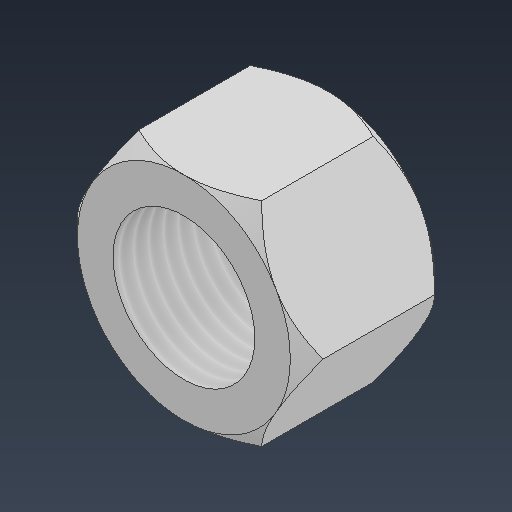
# Autodesk Inventor part: MCEN4000:T4
Saved by Autodesk Inventor 2021 (Build 250183000, 183)
## iProperties
Created: 2020-10-18
Part Number: MCEN4000:T4
Material: Generic
Document SubType Name: Modeling
Designer: Eugene Tang
Mass: 2.02151 g
Surface Area: 15.1772 cm^2
Volume: 2.02151 cm^3
Density: 1 g/cm^3
Appearance: Default
Description: NUT FASTENER
Author: Eugene Tang
Autodesk Inventor part; units mm, degrees
ref_plane "YZ Plane" through (0, 0, 0) normal (1, 0, 0) x (0, 1, 0)
ref_plane "XZ Plane" through (0, 0, 0) normal (0, 1, 0) x (-1, 0, 0)
ref_plane "XY Plane" through (0, 0, 0) normal (0, 0, 1) x (1, 0, 0)
sketch "Sketch1" plane through (0, 0, 0) normal (0, 0, 1) x (1, 0, 0)
  line L0 (10.3923, 0) -> (5.1962, -9)
  line L1 (5.1962, -9) -> (-5.1962, -9)
  line L2 (-5.1962, -9) -> (-10.3923, 0)
  line L3 (-10.3923, 0) -> (-5.1962, 9)
  line L4 (-5.1962, 9) -> (5.1962, 9)
  line L5 (5.1962, 9) -> (10.3923, 0)
  circle A0 centre (0, 0) radius 6
  dimension "d2" = 18
  dimension "d3" = 12
  constraints: 12 end point, 2 coincident, 1 centre point, 1 horizontal, 13 other
  measures "d2" distance between parallel lines of L3 L0
  measures "d3" diameter of A0
extrude "Extrusion2" add sketch "Sketch1" along normal blind 12.2
sketch "Sketch2" plane through (0, 0, 12.2) normal (0, 0, 1) x (1, 0, 0)
  circle A0 centre (0, 0) radius 6 construction
  circle A1 centre (0, 0) radius 9
  line L0 (-10.3923, 0) -> (-5.1962, -9) construction
  constraints: 1 centre point, 1 coincident, 1 tangent
extrude "Extrusion3" cut sketch "Sketch2" against normal up to surface (12.2 mm away) draft 45 keep common part
sketch "Sketch3" plane through (0, 0, 0) normal (0, 0, -1) x (-1, 0, 0)
  circle A0 centre (0, 0) radius 6 construction
  circle A1 centre (0, 0) radius 9
  line L0 (-5.1962, -9) -> (-10.3923, 0) construction
  constraints: 1 centre point, 1 coincident, 1 tangent
extrude "Extrusion4" cut sketch "Sketch3" against normal up to surface (12.2 mm away) draft 45 keep common part
thread "Thread1" size "M12x1.25" class "6H" standard "ISO Metric profile" full length
equation "\"d3\" = Screw_DIA"
equation "\"d19\" = 55deg"
equation "\"Sketch4_Pitch\" = 1.25"
equation "\"Screw_DIA\" = 12"
body "Solid2"
